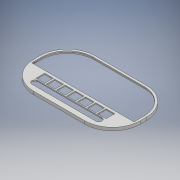
# Autodesk Inventor part: Game_ColoniesV2
Saved by Autodesk Inventor 2018 (Build 220112000, 112)
## iProperties
Created: 2021-04-22
Part Number: Game_ColoniesV2
Material: Generic
Document SubType Name: Modeling
Designer: Bradley
Density: 1 g/cm^3
Appearance: Default
Author: Bradley
Autodesk Inventor part; units mm, degrees
ref_plane "YZ Plane" through (0, 0, 0) normal (1, 0, 0) x (0, 1, 0)
ref_plane "XZ Plane" through (0, 0, 0) normal (0, 1, 0) x (-1, 0, 0)
ref_plane "XY Plane" through (0, 0, 0) normal (0, 0, 1) x (1, 0, 0)
sketch "Sketch1" plane through (0, 0, 0) normal (0, 0, 1) x (1, 0, 0)
  line L0 (-25, -30) -> (25, -30)
  line L1 (52, -3) -> (52, 3)
  line L2 (25, 30) -> (-25, 30)
  line L3 (-52, 3) -> (-52, -3)
  line L4 (-52, -30) -> (52, 30) construction
  line L5 (52, -30) -> (-52, 30) construction
  arc A0 (-25, 30) -> (-52, 3) centre (-25, 3) ccw
  arc A1 (52, 3) -> (25, 30) centre (25, 3) ccw
  arc A2 (25, -30) -> (52, -3) centre (25, -3) ccw
  arc A3 (-52, -3) -> (-25, -30) centre (-25, -3) ccw
  line L6 (-51.1, 3) -> (-51.1, -3)
  arc A4 (-51.1, -3) -> (-25, -29.1) centre (-25, -3) ccw
  line L7 (-25, -29.1) -> (25, -29.1)
  arc A5 (25, -29.1) -> (51.1, -3) centre (25, -3) ccw
  line L8 (51.1, -3) -> (51.1, 3)
  arc A6 (51.1, 3) -> (25, 29.1) centre (25, 3) ccw
  line L9 (25, 29.1) -> (-25, 29.1)
  arc A7 (-25, 29.1) -> (-51.1, 3) centre (-25, 3) ccw
  line L10 (-25, 28) -> (25, 28)
  arc A8 (50, 3) -> (25, 28) centre (25, 3) ccw
  line L11 (50, 3) -> (50, -7)
  line L12 (-50, -7) -> (-50, 3)
  arc A9 (-25, 28) -> (-50, 3) centre (-25, 3) ccw
  line L13 (-50, -7) -> (50, -7)
  line L14 (-34.85, -9.5) -> (-26.35, -9.5)
  line L15 (-26.35, -9.5) -> (-26.35, -18)
  line L16 (-26.35, -18) -> (-34.85, -18)
  line L17 (-34.85, -18) -> (-34.85, -9.5)
  line L18 (-24.85, -9.5) -> (-16.35, -9.5)
  line L19 (-24.85, -18) -> (-24.85, -9.5)
  line L20 (-16.35, -9.5) -> (-16.35, -18)
  line L21 (-16.35, -18) -> (-24.85, -18)
  line L22 (-14.85, -9.5) -> (-6.35, -9.5)
  line L23 (-14.85, -18) -> (-14.85, -9.5)
  line L24 (-6.35, -9.5) -> (-6.35, -18)
  line L25 (-6.35, -18) -> (-14.85, -18)
  line L26 (-4.85, -9.5) -> (3.65, -9.5)
  line L27 (-4.85, -18) -> (-4.85, -9.5)
  line L28 (3.65, -9.5) -> (3.65, -18)
  line L29 (3.65, -18) -> (-4.85, -18)
  line L30 (5.15, -9.5) -> (13.65, -9.5)
  line L31 (5.15, -18) -> (5.15, -9.5)
  line L32 (13.65, -9.5) -> (13.65, -18)
  line L33 (13.65, -18) -> (5.15, -18)
  line L34 (15.15, -9.5) -> (23.65, -9.5)
  line L35 (15.15, -18) -> (15.15, -9.5)
  line L36 (23.65, -9.5) -> (23.65, -18)
  line L37 (23.65, -18) -> (15.15, -18)
  line L38 (25.15, -9.5) -> (33.65, -9.5)
  line L39 (25.15, -18) -> (25.15, -9.5)
  line L40 (33.65, -9.5) -> (33.65, -18)
  line L41 (33.65, -18) -> (25.15, -18)
  line L42 (-31.85, -22) -> (30.65, -22) construction
  line L43 (-31.85, -25) -> (30.65, -25)
  line L44 (30.65, -19) -> (-31.85, -19)
  arc A10 (-31.85, -19) -> (-31.85, -25) centre (-31.85, -22) ccw
  arc A11 (30.65, -25) -> (30.65, -19) centre (30.65, -22) ccw
  point P0 (0, 0)
  point P1 (-0.6, -22)
  dimension "d0" = 104
  dimension "d1" = 60
  dimension "d2" = 27
  dimension "d3" = 58.2
  dimension "d4" = 2
  dimension "d5" = 23
  dimension "d6" = 8.5
  dimension "d9" = 10
  dimension "d14" = 20.5
  dimension "d15" = 17.15
  dimension "d16" = 62.5
  dimension "d17" = 6
  dimension "d18" = 5
  dimension "d19" = 20.15
  constraints: 92 end point, 24 point on circle, 13 tangent, 12 centre point, 8 parallel, 8 point on line, 5 horizontal, 4 perpendicular, 3 equal radius, 3 midpoint, 58 other
  measures "d0" distance of L5.end L4.end
  measures "d1" distance of L4.end L5.start
  measures "d2" radius of A0
  measures "d3" distance between parallel lines of L7 L9
  measures "d4" distance between parallel lines of L2 L10
  measures "d5" distance between parallel lines of L0 L13
  measures "d6" distance of L15.end L16.end
  measures "d9" distance of L14.start L18.start
  measures "d14" distance between parallel lines of L0 L14
  measures "d15" distance between parallel lines of L3 L17
  measures "d16" distance of L42.start L42.end
  measures "d17" diameter of A11
  measures "d18" distance between parallel lines of L0 L43
  measures "d19" distance from line of L3 L42.start
extrude "Extrusion1" add sketch "Sketch1" against normal blind 2 contours A3 L3 A0 L2 A1 L1 A2 L0
extrude "Extrusion2" add sketch "Sketch1" along normal blind 1 contours A3 L3 A0 L2 A1 L1 A2 L0 | A7 L9 A6 L8 A5 L7 A4 L6
body "Solid1"
